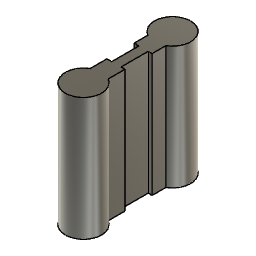
hinge 2 (Autodesk Fusion 360 design; units mm, degrees)
Autodesk Fusion 360 part; units mm, degrees
sketch "Sketch1" plane through (0, 0, 0) normal (0, 0, 1) x (1, 0, 0)
  circle A0 centre (0, 0) radius 2.5
  line L0 (-1.25, 2.1651) -> (-1.25, 10.1651)
  line L1 (1.25, 2.1651) -> (1.25, 10.1651)
  circle A1 centre (0, 12.3301) radius 2.5
  dimension "d1" = 5
  dimension "d3" = 2.5
  dimension "d4" = 1.25
  dimension "d5" = 5
  dimension "d6" = 8
  dimension "d7" = 8
  constraint coincident A0.centre origin
  constraint coincident A0 L0.start
  constraint vertical L0
  constraint coincident A0 L1.start
  constraint parallel L0 L1
  constraint coincident L0.end A1
  constraint coincident L1.end A1
  measures "d1" diameter of A0
  measures "d3" distance of L0 L1
  measures "d4" distance of A0.centre L1
  measures "d5" diameter of A1
  measures "d6" distance of L1.start L1.end
  measures "d7" distance of L0.start L0.end
extrude "Extrude1" add sketch "Sketch1" along normal blind 17
sketch "Sketch2" plane through (0, 0, 17) normal (0, 0, 1) x (-1, 0, 0)
  arc A0 (1.25, -2.1651) -> (-1.25, -2.1651) centre (0, 0) ccw
  line L0 (-1.25, -2.1651) -> (-1.25, -10.1651)
  arc A1 (-1.25, -10.1651) -> (1.25, -10.1651) centre (0, -12.3301) ccw
  line L1 (1.25, -10.1651) -> (1.25, -2.1651)
  line L2 (1.25, -8.2573) -> (-1.25, -8.2573)
  line L3 (-1.25, -8.2573) -> (-1.25, -4.505)
  line L4 (-1.25, -4.505) -> (1.25, -4.505)
  line L5 (1.25, -4.505) -> (1.25, -8.2573)
  line L6 (0.5809, -8.2573) -> (0.5809, -4.505)
  line L7 (-0.7066, -8.2573) -> (-0.7066, -4.505)
  constraint horizontal L2
  constraint vertical L3
  constraint horizontal L4
  constraint vertical L5
  constraint coincident L0 L3.end
  constraint coincident L1 L2.start
  constraint coincident L2 L6.start
  constraint coincident L4 L6.end
  constraint perpendicular L4 L6
  constraint coincident L2 L7.start
  constraint coincident L4 L7.end
  constraint perpendicular L4 L7
extrude "Extrude2" cut sketch "Sketch2" against normal blind 18 contours L1 L2 L4 L5 L6 | L0 L2 L3 L4 L7
